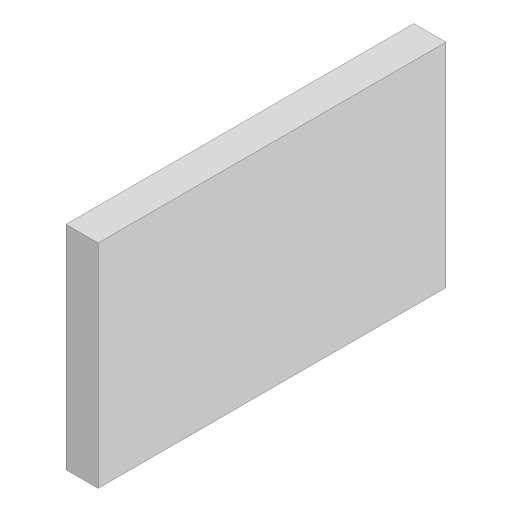
# Autodesk Inventor part: PANTALLA
Saved by Autodesk Inventor 2024 (Build 280153000, 153)
## iProperties
Created: 2024-07-01
Part Number: PANTALLA
Material: Generic
Document SubType Name: Modeling
Designer: Jhuliams
Density: 1 g/cm^3
Appearance: Default
Author: Jhuliams
Autodesk Inventor part; units mm, degrees
ref_plane "YZ Plane" through (0, 0, 0) normal (1, 0, 0) x (0, 1, 0)
ref_plane "XZ Plane" through (0, 0, 0) normal (0, 1, 0) x (-1, 0, 0)
ref_plane "XY Plane" through (0, 0, 0) normal (0, 0, 1) x (1, 0, 0)
sketch "Sketch1" plane through (0, 0, 0) normal (1, 0, 0) x (0, 1, 0)
  line L0 (165, 270) -> (-165, 270)
  line L1 (-165, 270) -> (-165, -270)
  line L2 (-165, -270) -> (165, -270)
  line L3 (165, -270) -> (165, 270)
  line L4 (165, 270) -> (-165, -270) construction
  line L5 (-165, 270) -> (165, -270) construction
  point P0 (0, 0)
  dimension "d0" = 330
  dimension "d1" = 540
  constraints: 12 end point, 2 midpoint, 2 parallel, 1 horizontal, 1 perpendicular
  measures "d0" distance of L2.end L1.end
  measures "d1" distance of L1.end L0.end
extrude "Extrusion1" add sketch "Sketch1" along normal blind 50
body "Solid1"
